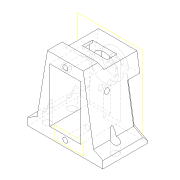
# Autodesk Inventor part: servo_clamp
Saved by Autodesk Inventor 2014 (Build 180170000, 170)
## iProperties
Created: 2015-05-30
Part Number: servo_clamp
Material: Generic
Document SubType Name: Modeling
Designer: Martin
Density: 1 g/cm^3
Appearance: Default
Author: Martin
Autodesk Inventor part; units mm, degrees
ref_plane "YZ Plane" through (0, 0, 0) normal (1, 0, 0) x (0, 1, 0)
ref_plane "XZ Plane" through (0, 0, 0) normal (0, 1, 0) x (-1, 0, 0)
ref_plane "XY Plane" through (0, 0, 0) normal (0, 0, 1) x (1, 0, 0)
ref_plane "Work Plane1" through (14.3392, -46.1241, 0) normal (0, -1, 0) x (-1, 0, 0)
sketch "sk_main" plane through (14.3392, -46.1241, 0) normal (0, -1, 0) x (-1, 0, 0)
  line L0 (-22.1702, 0) -> (47.1015, 0) projected
  line L1 (0.3, -25.8) -> (-11.3, -25.8) construction
  line L2 (-5.5, -25.8) -> (-5.5, 0) construction
  line L3 (0.8, 0) -> (0.8, -26.3)
  line L4 (0.8, -26.3) -> (-11.8, -26.3)
  line L5 (-11.8, -26.3) -> (-11.8, 0)
  line L6 (6.8, 0) -> (2.3, -27.3)
  line L7 (2.3, -27.3) -> (-13.3, -27.3)
  line L8 (-13.3, -27.3) -> (-17.8, 0)
  line L9 (5.9758, -5) -> (9.8, -3)
  line L10 (9.8, -3) -> (9.8, 0)
  line L11 (-16.9758, -5) -> (-20.8, -3)
  line L12 (-20.8, -3) -> (-20.8, 0)
  line L13 (5.9758, -5) -> (-16.9758, -5) construction
  line L14 (9.8, -3) -> (-20.8, -3) construction
  line L15 (-11.8, -4.2) -> (0.8, -4.2)
  line L16 (0.8, -4.2) -> (0.8, 0)
  line L17 (0.8, 0) -> (-11.8, 0)
  line L18 (-11.8, 0) -> (-11.8, -4.2)
  line L19 (-5.5, -4.2) -> (-5.5, 0) construction
  circle A0 centre (-5.5, -2.5) radius 1
  line L20 (-13.3, -27.3) -> (-12.7725, -30.5)
  line L21 (-12.7725, -30.5) -> (1.7725, -30.5)
  line L22 (1.7725, -30.5) -> (2.3, -27.3)
  line L23 (-5.5, -26.3) -> (-5.5, -30.5) construction
  circle A1 centre (-5.5, -28) radius 1
  point P0 (14.3392, 0)
  dimension "d0" = 1
  dimension "d1" = 0.5
  dimension "d2" = 0.5
  dimension "d3" = 1.5
  dimension "d4" = 6
  dimension "d24" = 3
  dimension "d25" = 2
  dimension "d26" = 3
  dimension "d27" = 3
  dimension "d51" = 4.2
  dimension "d52" = 2
  dimension "d53" = 2.5
  dimension "d54" = 4.2
  dimension "d55" = 2.5
  constraints: 46 end point, 8 perpendicular, 5 point on line, 4 midpoint, 4 vertical, 3 parallel, 3 symmetric about line, 2 centre point, 2 collinear, 1 horizontal, 12 other
  measures "d0" distance between parallel lines of L7 L4
  measures "d1" distance from line of L5 L1.end
  measures "d2" distance from line of L1.end L4
  measures "d3" horizontal distance of L6.end L3.end
  measures "d4" distance of L3.start L6.start
  measures "d24" distance of L6.start L10.end
  measures "d25" distance between parallel lines of L14 L13
  measures "d26" distance of L9.end L10.end
  measures "d27" distance of L8.end L12.end
  measures "d51" distance between parallel lines of L17 L15
  measures "d52" diameter of A0
  measures "d54" distance between parallel lines of L21 L4
  measures "d55" distance from line of L21 A1.centre
extrude "ext_maincage" add sketch "sk_main" against normal blind 16 contours L0 L8 L11 L12 | L0 L5 L4 L3 L6 L7 A1 L8 | L0 L3 L15 L5 | L0 L10 L9 L6 | A1 L7 | A0 picked at (-5.4791, -27.1545)
sketch "Sketch2" plane through (14.3392, -30.1241, 0) normal (0, 1, 0) x (1, 0, 0)
  line L0 (-0.8, -26.3) -> (-0.8, -4.2) projected
  line L1 (-2.3, -27.3) -> (13.3, -27.3) projected
  line L2 (11.8, -4.2) -> (11.8, -26.3) projected
  line L3 (11.8, -26.3) -> (-0.8, -26.3) projected
  circle A0 centre (5.5, -20) radius 5.5
  circle A1 centre (5.5, -20) radius 7.3
  line L4 (-0.8, 0) -> (-0.8, -16.3122)
  line L5 (9.1878, -26.3) -> (11.8, -26.3)
  line L6 (11.8, -23.6878) -> (11.8, -26.3)
  line L7 (-0.8, 0) -> (11.8, 0)
  line L8 (11.8, 0) -> (11.8, -16.3122)
  line L9 (-0.8, -16.3122) -> (-0.8, 0)
  line L10 (20.8, 0) -> (-9.8, 0) projected
  line L11 (-9.8, 0) -> (-9.8, -3) projected
  line L12 (-9.8, -3) -> (-5.9758, -5) projected
  line L13 (-5.9758, -5) -> (-2.3, -27.3) projected
  line L14 (-2.3, -27.3) -> (13.3, -27.3) projected
  line L15 (13.3, -27.3) -> (16.9758, -5) projected
  line L16 (16.9758, -5) -> (20.8, -3) projected
  line L17 (20.8, -3) -> (20.8, 0) projected
  line L18 (11.8, -4.2) -> (11.8, -26.3) projected
  line L19 (11.8, -26.3) -> (-0.8, -26.3) projected
  line L20 (-0.8, -26.3) -> (-0.8, -4.2) projected
  line L21 (-0.8, -4.2) -> (11.8, -4.2) projected
  line L22 (-0.8, -23.6878) -> (-0.8, -26.3)
  line L23 (1.8122, -26.3) -> (-0.8, -26.3)
  arc A2 (-0.8, -23.6878) -> (1.8122, -26.3) centre (5.5, -20) ccw
  arc A3 (9.1878, -26.3) -> (11.8, -23.6878) centre (5.5, -20) ccw
  line L24 (9.1878, -26.3) -> (11.8, -26.3)
  line L25 (11.8, -26.3) -> (11.8, -23.6878)
  line L26 (-9.8, 0) -> (-9.8, -3) projected
  line L27 (-9.8, -3) -> (-5.9758, -5) projected
  line L28 (-5.9758, -5) -> (-2.3, -27.3) projected
  line L29 (13.3, -27.3) -> (16.9758, -5) projected
  line L30 (20.8, -3) -> (20.8, 0) projected
  line L31 (-0.8, 0) -> (-9.8, 0)
  line L32 (-9.8, 0) -> (-9.8, -3)
  line L33 (-9.8, -3) -> (-5.9758, -5)
  line L34 (-5.9758, -5) -> (-2.3, -27.3)
  line L35 (-2.3, -27.3) -> (5.5, -27.3)
  line L36 (5.5, -27.3) -> (13.3, -27.3)
  line L37 (13.3, -27.3) -> (16.9758, -5)
  line L38 (16.9758, -5) -> (20.8, -3)
  line L39 (20.8, 0) -> (20.8, -3)
  line L40 (20.8, 0) -> (11.8, 0)
  point P0 (-14.3392, 0)
  dimension "d7" = 11
  constraints: 40 end point, 11 collinear, 10 point on circle, 6 perpendicular, 5 point on line, 4 centre point, 2 coincident, 2 concentric, 2 tangent, 1 midpoint, 1 parallel, 1 other
  measures "d7" diameter of A0
extrude "ext_backhousing" add sketch "Sketch2" along normal blind 4.3
sketch "Sketch3" plane through (14.3392, -25.8241, 0) normal (0, 1, 0) x (1, 0, 0)
  line L0 (17.8, 0) -> (-6.8, 0) projected
  line L1 (-6.8, 0) -> (-2.3, -27.3) projected
  line L2 (-2.3, -27.3) -> (13.3, -27.3) projected
  line L3 (13.3, -27.3) -> (17.8, 0) projected
  circle A0 centre (5.5, -20) radius 2.5
  circle A1 centre (5.5, -20) radius 5.5 projected
  line L4 (20.8, 0) -> (-9.8, 0) projected
  line L5 (-2.3, -27.3) -> (13.3, -27.3) projected
  line L6 (16.9758, -5) -> (20.8, -3) projected
  line L7 (-9.8, 0) -> (-9.8, -3) projected
  line L8 (-9.8, -3) -> (-5.9758, -5) projected
  line L9 (-5.9758, -5) -> (-2.3, -27.3) projected
  line L10 (13.3, -27.3) -> (16.9758, -5) projected
  line L11 (20.8, -3) -> (20.8, 0) projected
  point P0 (-0.8, 0)
  point P1 (-14.3392, 0)
  dimension "d10" = 5
  constraints: 1 centre point
  measures "d10" diameter of A0
extrude "ext_backcover" add sketch "Sketch3" along normal blind 1 contours L3 L2 L1 L0 | L4 L11 L6 L3 | L1 L8 L7 L4 | A1
sketch "Sketch4" plane through (14.3392, -24.8241, 0) normal (0, 1, 0) x (1, 0, 0)
  circle A0 centre (5.5, -20) radius 2.5 projected
  line L0 (5.5, 0) -> (5.5, -17.5)
  line L1 (5.5, -15) -> (2.6132, -10)
  line L2 (2.6132, -10) -> (2.6132, 0)
  line L3 (20.8, 0) -> (-9.8, 0) projected
  line L4 (20.8, -3) -> (20.8, 0) projected
  line L5 (8, -20) -> (14.5033, -20)
  line L6 (-2.3, -27.3) -> (13.3, -27.3) projected
  line L7 (16.9758, -5) -> (20.8, -3) projected
  circle A1 centre (5.5, -20) radius 2.5
  line L8 (16.9758, -5) -> (20.8, -3)
  line L9 (20.8, -3) -> (20.8, 0)
  line L10 (20.8, 0) -> (5.5, 0)
  line L11 (13.3, -27.3) -> (16.9758, -5) projected
  line L12 (14.5033, -20) -> (16.9758, -5)
  line L13 (20.8, -3) -> (20.8, 0) projected
  line L14 (2.6132, 0) -> (5.5, 0)
  point P0 (-14.3392, 0)
  dimension "d22" = 30
  dimension "d23" = 10
  dimension "d28" = 5
  constraints: 18 end point, 3 collinear, 3 perpendicular, 2 line through centre, 2 point on circle, 2 point on line, 1 centre point, 1 coincident, 1 concentric, 1 midpoint, 1 parallel
  measures "d22" angle of L0 L1
  measures "d23" distance of L1.end L2.end
  measures "d28" vertical distance of L1.end L1.start
extrude "ext_cut_backcutway" cut sketch "Sketch4" against normal blind 3 contours A0 L0 L3 L4 L7 L11 L5 | L1 L2 L3 L0
chamfer "Chamfer3" distance 2 angle 45 2 edges at (30.0788, -27.8241, 12.5) (33.2272, -27.8241, 4)
ref_plane "back_plane" through (14.3392, -24.8241, 0) normal (0, 1, 0) x (1, 0, 0)
sketch "Sketch6" plane through (0, 0, 0) normal (0, 0, 1) x (1, 0, 0)
  line L0 (35.1392, -46.1241) -> (35.1392, -30.1241) projected
  circle A0 centre (32.1392, -38.1241) radius 1.5
  line L1 (33.6392, -38.1241) -> (35.1392, -38.1241)
  line L2 (32.1392, -38.1241) -> (33.6392, -38.1241) construction
  line L3 (4.5392, -46.1241) -> (4.5392, -30.1241) projected
  line L4 (4.5392, -46.1241) -> (4.5392, -30.1241) projected
  circle A1 centre (7.5392, -31.1241) radius 1.5
  circle A2 centre (7.5392, -41.1241) radius 1.5
  line L5 (7.5392, -31.1241) -> (7.5392, -41.1241) construction
  line L6 (7.5392, -41.1241) -> (6.0392, -41.1241) construction
  line L7 (7.5392, -31.1241) -> (6.0392, -31.1241) construction
  line L8 (4.5392, -31.1241) -> (6.0392, -31.1241)
  line L9 (4.5392, -41.1241) -> (6.0392, -41.1241)
  line L10 (35.1392, -46.1241) -> (35.1392, -30.1241) projected
  point P0 (0, 0)
  point P1 (4.5392, -24.8241)
  point P2 (35.1392, -27.8241)
  point P3 (4.5392, -26.8241)
  point P4 (35.1392, -29.8241)
  dimension "d38" = 3
  dimension "d40" = 1.5
  dimension "d43" = 10
  dimension "d44" = 5
  constraints: 14 end point, 4 parallel, 3 perpendicular, 2 horizontal alignment, 2 point on circle, 2 point on line, 1 centre point, 1 collinear, 1 midpoint, 5 other
  measures "d40" distance of L1.start L1.end
  measures "d43" distance of L5.start L5.end
  measures "d44" distance from line of L9 L3.start
extrude "ext_cut_bottomscrews" cut sketch "Sketch6" along normal through all
sketch "Sketch7" plane through (26.1392, -46.1241, 0) normal (-1, 0, 0) x (0, 0, 1)
  line L0 (26.3, 0) -> (26.3, 16) projected
  line L1 (26.3, 8) -> (0, 8) construction
  circle A0 centre (20.3, 8) radius 1
  point P0 (0, 46.1241)
  dimension "d47" = 2
  dimension "d48" = 6
  constraints: 2 end point, 1 centre point, 1 midpoint, 1 point on line
  measures "d47" diameter of A0
  measures "d48" distance from line of L0 A0.centre
extrude "ext_cut_lateralscrews" cut sketch "Sketch7" along normal through all both and the other way through all
sketch "sk_fixation&screws" plane through (14.3392, -46.1241, 0) normal (0, -1, 0) x (1, 0, 0)
  line L0 (13.3, 27.3) -> (-2.3, 27.3) projected
  line L1 (-0.8, 26.3) -> (11.8, 26.3) projected
  line L2 (-1.7725, 30.5) -> (-2.3, 27.3) projected
  line L3 (12.7725, 30.5) -> (-1.7725, 30.5) projected
  line L4 (13.3, 27.3) -> (12.7725, 30.5) projected
  circle A0 centre (5.5, 2.5) radius 1 projected
  circle A1 centre (5.5, 28) radius 1 projected
  point P0 (-14.3392, 0)
extrude "ext_top_fixationblock" add sketch "sk_fixation&screws" against normal blind 8 contours L0 A1 L2 L3 L4 | L0 A1 picked at (5.5339, 27.8649)
extrude "ext_cut_fixationscrews" cut sketch "sk_fixation&screws" against normal blind 9 contours A1 L0 | L0 A1 | A0
chamfer "Chamfer4" distance 3.2 distance2 2 1 edges at (19.8392, -38.1241, 30.5) measured on face at (19.8392, -38.1241, 30)
sketch "Sketch9" plane through (12.0392, -24.8241, 27.3) normal (0, 0, 1) x (1, 0, 0)
  line L0 (14.1, -5.3) -> (1.5, -5.3) projected
  line L1 (7.8, -5.3) -> (7.8, -9.3) construction
  line L2 (2.8, -9.3) -> (12.8, -9.3)
  line L3 (12.8, -9.3) -> (12.8, -5.3)
  line L4 (12.8, -5.3) -> (2.8, -5.3)
  line L5 (2.8, -5.3) -> (2.8, -9.3)
  line L6 (2.8, -9.3) -> (12.8, -5.3) construction
  line L7 (12.8, -9.3) -> (2.8, -5.3) construction
  point P0 (-12.0392, 24.8241)
  point P1 (7.8, -7.3)
  dimension "d63" = 4
  dimension "d64" = 10
  constraints: 14 end point, 4 midpoint, 2 parallel, 2 perpendicular, 1 horizontal, 1 point on line
  measures "d63" distance of L2.end L3.end
  measures "d64" distance of L3.end L4.end
extrude "Extrusion10" cut sketch "Sketch9" against normal up to surface (1 mm away)
equation "\"d7\" = linact_bearing_diameter"
equation "\"d8\" = linact_bearing_thickness"
equation "\"d38\" = screw_m3_bore_selfthreading"
equation "\"d47\" = screw_m2_bore_selfthreading"
equation "\"linact_bearing_diameter\" = 11"
equation "\"linact_bearing_thickness\" = 4.3"
equation "\"screw_m3_bore_selfthreading\" = 3"
equation "\"screw_m2_bore_selfthreading\" = 2"
body "Solid1"
